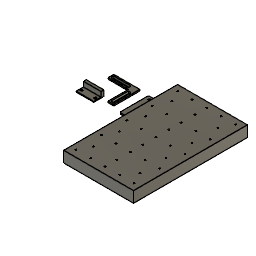
Spoilboard (Autodesk Fusion 360 design; units mm, degrees)
Autodesk Fusion 360 part; units mm, degrees
note: some values were not read from the file. Set by a fixed rule: which sketch regions a step uses.
sketch "Sketch1" plane through (0, 0, 0) normal (0, 1, 0) x (1, 0, 0)
  line L0 (0, 0) -> (60, 0)
  line L1 (60, 0) -> (60, -80)
  line L2 (60, -80) -> (0, -80)
  line L3 (0, -80) -> (0, 0)
  line L4 (40, -80) -> (0, -40)
  line L5 (60, -80) -> (50, -80)
  line L6 (50, -40) -> (60, -40)
  line L7 (60, -40) -> (60, -80)
  circle A0 centre (50, -70) radius 2.5
  circle A1 centre (50, -50) radius 2.5
  line L8 (0, 0) -> (55, 0)
  line L9 (55, 0) -> (55, -10)
  line L10 (55, -10) -> (0, -10)
  line L11 (0, -10) -> (0, 0)
  line L12 (0, 0) -> (55, 0)
  line L13 (55, 0) -> (55, -30)
  line L14 (55, -30) -> (0, -30)
  line L15 (0, -30) -> (0, 0)
  circle A2 centre (20, -30) radius 1.55
  circle A3 centre (40, -30) radius 1.55
  circle A4 centre (20, -10) radius 1.55
  circle A5 centre (40, -10) radius 1.55
  dimension "d1" = 60
  dimension "d2" = 80
  dimension "d3" = 20
  dimension "d4" = 40
  dimension "d5" = 5
  dimension "d6" = 5
  dimension "d7" = 10
  dimension "d8" = 30
  dimension "d9" = 3.1
  dimension "d10" = 3.1
  dimension "d11" = 3.1
  dimension "d12" = 3.1
  dimension "d13" = 20
  dimension "d14" = 20
  dimension "d15" = 20
  dimension "d16" = 20
  constraint horizontal L0
  constraint vertical L1
  constraint horizontal L2
  constraint vertical L3
  constraint coincident L0.start L3.end
  constraint coincident L2 L4.start
  constraint coincident L3 L4.end
  constraint horizontal L5
  constraint horizontal L6
  constraint vertical L7
  constraint horizontal L8
  constraint vertical L9
  constraint horizontal L10
  constraint vertical L11
  constraint horizontal L12
  constraint vertical L13
  constraint horizontal L14
  constraint vertical L15
  constraint coincident L14 A2.centre
  constraint coincident L14 A3.centre
  constraint coincident L10 A4.centre
  constraint coincident L10 A5.centre
  measures "d1" distance of L0.start L0.end
  measures "d2" distance of L0.start L2.end
  measures "d3" distance of L1.end L4.start
  measures "d4" distance of L0 L4.end
  measures "d5" diameter of A0
  measures "d6" diameter of A1
  measures "d7" distance of L0.start L10.end
  measures "d8" distance of L0.start L14.end
  measures "d9" diameter of A2
  measures "d10" diameter of A3
  measures "d11" diameter of A4
  measures "d12" diameter of A5
  measures "d13" distance of L15 A4.centre
  measures "d14" distance of L1 A5.centre
  measures "d15" distance of L1 A3.centre
  measures "d16" distance of L3 A2.centre
extrude "Extrude1" add sketch "Sketch1" against normal blind 10 contours L0 L3 L8 L9 L10 L11 L12 L13 L15 A4 A5 | L0 L1 L2 L3 L4 L5 L7 L9 L13 L14 A2 A3 | L3 L10 L13 L14 L15 A2 A3 A4 A5 makes body 1
sketch "Sketch2" plane through (0, -10, 0) normal (0, -1, 0) x (1, 0, 0)
  circle A0 centre (40, 30) radius 1.55
  circle A1 centre (20, 30) radius 1.55
  circle A2 centre (50, 70) radius 2.5
  circle A3 centre (20, 10) radius 1.55
  circle A4 centre (50, 50) radius 2.5
  circle A5 centre (40, 10) radius 1.55
  line L0 (0, 40) -> (0, 0)
  line L1 (0, 0) -> (60, 0)
  line L2 (60, 0) -> (60, 80)
  line L3 (60, 80) -> (40, 80)
  line L4 (40, 80) -> (0, 40)
  circle A6 centre (20, 30) radius 3
  circle A7 centre (40, 30) radius 3
  circle A8 centre (40, 10) radius 3
  circle A9 centre (20, 10) radius 3
  dimension "d19" = 6
  dimension "d20" = 6
  dimension "d21" = 6
  dimension "d22" = 6
  constraint concentric A1 A6
  constraint concentric A0 A7
  constraint concentric A5 A8
  constraint concentric A3 A9
  measures "d19" diameter of A6
  measures "d20" diameter of A7
  measures "d21" diameter of A8
  measures "d22" diameter of A9
extrude "Extrude2" cut sketch "Sketch2" against normal blind 6.5 contours A6 | A7 | A8 | A9 bodies 1
ref_plane "WorkPlane1" through (-10, -5, 20) normal (-1, 0, 0) x (0, 0, -1)
sketch "Sketch3" plane through (0, 0, 0) normal (0, 0, 1) x (1, 0, 0)
  line L0 (0, 0) -> (241, 0)
  line L1 (241, 0) -> (241, -393)
  line L2 (241, -393) -> (0, -393)
  line L3 (0, -393) -> (0, 0)
  dimension "d30" = 393
  dimension "d31" = 241
  constraint horizontal L0
  constraint vertical L1
  constraint horizontal L2
  constraint vertical L3
  constraint coincident L0.start L3.end
  measures "d30" distance of L0.start L2.end
  measures "d31" distance of L0.start L0.end
extrude "Extrude4" add sketch "Sketch3" along normal blind 38 separate body makes body 2
sketch "Sketch4" plane through (0, 0, 38) normal (0, 0, 1) x (-1, 0, 0)
  line L0 (0, 393) -> (-241, 393)
  line L1 (-241, 393) -> (-241, 0)
  line L2 (-241, 0) -> (0, 0)
  line L3 (0, 0) -> (0, 393)
  point P0 (-220, 20)
  point P1 (-170, 20)
  point P2 (-120, 20)
  point P3 (-70, 20)
  point P4 (-20, 20)
  point P5 (-220, 107.5)
  point P6 (-170, 107.5)
  point P7 (-120, 107.5)
  point P8 (-70, 107.5)
  point P9 (-20, 107.5)
  point P10 (-220, 195)
  point P11 (-170, 195)
  point P12 (-120, 195)
  point P13 (-70, 195)
  point P14 (-20, 195)
  point P15 (-220, 282.5)
  point P16 (-170, 282.5)
  point P17 (-120, 282.5)
  point P18 (-70, 282.5)
  point P19 (-20, 282.5)
  point P20 (-220, 370)
  point P21 (-170, 370)
  point P22 (-120, 370)
  point P23 (-70, 370)
  point P24 (-20, 370)
  point P25 (-200, 60)
  point P26 (-120, 60)
  point P27 (-40, 60)
  point P28 (-200, 150)
  point P29 (-120, 150)
  point P30 (-40, 150)
  point P31 (-200, 240)
  point P32 (-120, 240)
  point P33 (-40, 240)
  point P34 (-200, 330)
  point P35 (-120, 330)
  point P36 (-40, 330)
  dimension "d36" = 200
  dimension "d37" = 350
  dimension "d40" = 160
  dimension "d41" = 270
hole "Hole1" at (70, -370, 38) at (20, -370, 38) at (40, -330, 38) at (120, -370, 38) at (170, -370, 38) at (220, -370, 38) at (200, -330, 38) at (120, -330, 38) at (220, -282.5, 38) at (170, -282.5, 38) at (20, -282.5, 38) at (70, -282.5, 38) at (120, -282.5, 38) at (120, -240, 38) at (200, -240, 38) at (40, -240, 38) at (20, -195, 38) at (70, -195, 38) at (120, -195, 38) at (170, -195, 38) at (220, -195, 38) at (200, -150, 38) at (120, -150, 38) at (40, -150, 38) at (20, -107.5, 38) at (70, -107.5, 38) at (120, -107.5, 38) at (170, -107.5, 38) at (220, -107.5, 38) at (200, -60, 38) at (120, -60, 38) at (40, -60, 38) at (20, -20, 38) at (70, -20, 38) at (120, -20, 38) at (170, -20, 38) at (220, -20, 38) direction (0, 0, -1) diameter 5 depth 38 tip angle 118 bodies 2
sketch "Sketch5" plane through (0, 0, 38) normal (0, 0, 1) x (-1, 0, 0)
  circle A0 centre (-170, 20) radius 2.5
  circle A1 centre (-70, 20) radius 2.5
  circle A2 centre (-40, 60) radius 2.5
  circle A3 centre (-200, 60) radius 2.5
  circle A4 centre (-170, 107.5) radius 2.5
  circle A5 centre (-70, 107.5) radius 2.5
  circle A6 centre (-40, 150) radius 2.5
  circle A7 centre (-200, 150) radius 2.5
  circle A8 centre (-170, 195) radius 2.5
  circle A9 centre (-70, 195) radius 2.5
  circle A10 centre (-40, 240) radius 2.5
  circle A11 centre (-120, 240) radius 2.5
  circle A12 centre (-70, 282.5) radius 2.5
  circle A13 centre (-170, 282.5) radius 2.5
  circle A14 centre (-120, 330) radius 2.5
  circle A15 centre (-220, 370) radius 2.5
  circle A16 centre (-120, 370) radius 2.5
  circle A17 centre (-20, 370) radius 2.5
  circle A18 centre (-70, 370) radius 2.5
  circle A19 centre (-40, 330) radius 2.5
  circle A20 centre (-170, 370) radius 2.5
  circle A21 centre (-200, 330) radius 2.5
  circle A22 centre (-220, 282.5) radius 2.5
  circle A23 centre (-20, 282.5) radius 2.5
  circle A24 centre (-120, 282.5) radius 2.5
  circle A25 centre (-200, 240) radius 2.5
  circle A26 centre (-20, 195) radius 2.5
  circle A27 centre (-120, 195) radius 2.5
  circle A28 centre (-220, 195) radius 2.5
  circle A29 centre (-120, 150) radius 2.5
  circle A30 centre (-20, 107.5) radius 2.5
  circle A31 centre (-120, 107.5) radius 2.5
  circle A32 centre (-220, 107.5) radius 2.5
  circle A33 centre (-120, 60) radius 2.5
  circle A34 centre (-20, 20) radius 2.5
  circle A35 centre (-120, 20) radius 2.5
  circle A36 centre (-220, 20) radius 2.5
  line L0 (0, 393) -> (-241, 393)
  line L1 (-241, 393) -> (-241, 0)
  line L2 (-241, 0) -> (0, 0)
  line L3 (0, 0) -> (0, 393)
  line L4 (80, 100) -> (80, 30)
  line L5 (80, 30) -> (100, 30)
  line L6 (100, 50) -> (100, 120)
  line L7 (100, 120) -> (80, 120)
  line L8 (80, 120) -> (80, 100)
  line L9 (100, 50) -> (170, 50)
  line L10 (100, 30) -> (170, 30)
  line L11 (170, 30) -> (170, 50)
  dimension "d46" = 90
  constraint vertical L4
  constraint perpendicular L4 L5
  constraint perpendicular L5 L6
  constraint perpendicular L6 L7
  constraint perpendicular L7 L8
  constraint perpendicular L6 L9
  constraint perpendicular L6 L10
  constraint perpendicular L10 L11
  measures "d46" distance of L4 L11
sketch "Sketch7" plane through (0, 0, 38) normal (0, 0, 1) x (-1, 0, 0)
  line L0 (85, 115) -> (95, 115)
  line L1 (95, 115) -> (95, 55)
  line L2 (95, 55) -> (85, 55)
  line L3 (85, 55) -> (85, 115)
  line L4 (105, 45) -> (165, 45)
  line L5 (165, 45) -> (165, 35)
  line L6 (165, 35) -> (105, 35)
  line L7 (105, 35) -> (105, 45)
  constraint horizontal L0
  constraint vertical L1
  constraint horizontal L2
  constraint vertical L3
  constraint horizontal L4
  constraint vertical L5
  constraint horizontal L6
  constraint vertical L7
extrude "Extrude9" add sketch "Sketch5" along normal blind 5 separate body contours L4 L5 L6 L7 L8 L9 L10 L11 makes body 3
extrude "Extrude10" cut sketch "Sketch7" along normal blind 20 bodies 3
draft "Draft1" angle 30 neutral plane through (0, 0, 43) pull (0, 0, 1) 8 faces at (-85, -75, 39.6667) (-105, -38.3333, 39.6667) (-95, -95, 39.6667) (-165, -41.6667, 39.6667) (-88.3333, -115, 39.6667) (-125, -45, 39.6667) (-145, -35, 39.6667) (-91.6667, -55, 39.6667) on bodies 3
move_body "Move7" bodies 3 to x (1, 0, 0) y (0, 1, 0) z (0, 0, 1) at (0, -20, -34.641)
sketch "Sketch8" plane through (0, 0, 0) normal (0, 0, 1) x (1, 0, 0)
  line L0 (-45, -50) -> (-25, -50)
  line L1 (-20, -55) -> (-20, -61.8388)
  line L2 (-37.6229, -150) -> (-45, -150)
  line L3 (-50, -145) -> (-50, -55)
  spline S0 degree 5 poles (-22.4081, -66.1145) (-22.6473, -66.2595) (-23.5601, -66.8506) (-25.0379, -68.0682) (-26.8635, -70.273) (-28.7085, -74.0094) (-30.1195, -79.4806) (-30.8706, -86.0261) (-31.077, -93.4328) (-30.8971, -101.4083) (-30.5136, -109.6167) (-30.1163, -117.7095) (-29.8841, -125.3579) (-29.9696, -132.2821) (-30.4781, -138.2915) (-31.2767, -142.3725) (-32.1097, -144.9675) (-32.7761, -146.499) (-33.1491, -147.2333) (-33.1747, -147.2833) knots 0.043571 0.043571 0.043571 0.043571 0.043571 0.043571 0.066667 0.133333 0.2 0.266667 0.333333 0.4 0.466667 0.533333 0.6 0.666667 0.733333 0.8 0.866667 0.933333 0.938232 0.938232 0.938232 0.938232 0.938232 0.938232
  arc A0 (-50, -145) -> (-45, -150) centre (-45, -145) ccw
  arc A1 (-37.6229, -150) -> (-33.1747, -147.2833) centre (-37.6229, -145) ccw
  arc A2 (-22.4081, -66.1145) -> (-20, -61.8388) centre (-25, -61.8388) ccw
  arc A3 (-20, -55) -> (-25, -50) centre (-25, -55) ccw
  arc A4 (-45, -50) -> (-50, -55) centre (-45, -55) ccw
  circle A5 centre (-36.5, -62) radius 2.5
  point P0 (-30, -80)
  point P1 (-30, -130)
  dimension "d61" = 5
  dimension "d62" = 5
  constraint horizontal L0
  constraint vertical L1
  constraint horizontal L2
  constraint vertical L3
  constraint tangent L2 A0
  constraint tangent L3 A0
  constraint tangent S0 A1
  constraint tangent L2 A1
  constraint equal A0 A1
  constraint tangent S0 A2
  constraint tangent L1 A2
  constraint equal A0 A2
  constraint tangent L0 A3
  constraint tangent L1 A3
  constraint equal A0 A3
  constraint tangent L0 A4
  constraint tangent L3 A4
  constraint equal A0 A4
  measures "d61" radius of A0
  measures "d62" diameter of A5
extrude "Extrude11" add sketch "Sketch8" along normal blind 5 separate body makes body 4
sketch "Sketch9" plane through (0, 0, 5) normal (0, 0, 1) x (-1, 0, 0)
  circle A0 centre (36.5, 62) radius 2.5
  arc A1 (20, 55) -> (25, 50) centre (25, 55) ccw
  line L0 (25, 50) -> (45, 50)
  arc A2 (45, 50) -> (50, 55) centre (45, 55) ccw
  line L1 (50, 55) -> (50, 145)
  arc A3 (50, 145) -> (45, 150) centre (45, 145) ccw
  line L2 (45, 150) -> (37.6229, 150)
  arc A4 (37.6229, 150) -> (33.1747, 147.2833) centre (37.6229, 145) ccw
  spline S0 degree 5 poles (33.1747, 147.2833) (33.1491, 147.2333) (32.7761, 146.499) (32.1097, 144.9675) (31.2767, 142.3725) (30.4781, 138.2915) (29.9696, 132.2821) (29.8841, 125.3579) (30.1163, 117.7095) (30.5136, 109.6167) (30.8971, 101.4083) (31.077, 93.4328) (30.8706, 86.0261) (30.1195, 79.4806) (28.7085, 74.0094) (26.8635, 70.273) (25.0379, 68.0682) (23.5601, 66.8506) (22.6473, 66.2595) (22.4081, 66.1145) knots -0.938232 -0.938232 -0.938232 -0.938232 -0.938232 -0.938232 -0.933333 -0.866667 -0.8 -0.733333 -0.666667 -0.6 -0.533333 -0.466667 -0.4 -0.333333 -0.266667 -0.2 -0.133333 -0.066667 -0.043571 -0.043571 -0.043571 -0.043571 -0.043571 -0.043571
  arc A5 (22.4081, 66.1145) -> (20, 61.8388) centre (25, 61.8388) ccw
  line L3 (20, 61.8388) -> (20, 55)
  circle A6 centre (36.5, 62.0016) radius 3.5
  dimension "d65" = 7
  measures "d65" diameter of A6
extrude "Extrude12" cut sketch "Sketch9" against normal blind 2.5 contours A6 bodies 4
sketch "Sketch10" plane through (0, 0, 0) normal (0, 0, 1) x (1, 0, 0)
  line L0 (-135, -160) -> (-190, -160)
  line L1 (-190, -160) -> (-190, -125)
  line L2 (-190, -125) -> (-135, -125)
  line L3 (-135, -125) -> (-135, -160)
  line L4 (-135, -135) -> (-190, -135)
  line L5 (-190, -135) -> (-190, -160)
  line L6 (-190, -160) -> (-135, -160)
  line L7 (-135, -160) -> (-135, -135)
  constraint horizontal L0
  constraint vertical L1
  constraint horizontal L2
  constraint vertical L3
  constraint horizontal L4
  constraint vertical L5
  constraint horizontal L6
  constraint vertical L7
  constraint coincident L3 L4.start
extrude "Extrude13" add sketch "Sketch10" along normal blind 3 separate body contours L0 L1 L3 L4 L5 L6 L7 makes body 5
extrude "Extrude14" add sketch "Sketch10" along normal blind 15 contours L1 L2 L3 L4 bodies 5
sketch "Sketch11" plane through (0, 0, 3) normal (0, 0, 1) x (-1, 0, 0)
  line L0 (135, 160) -> (135, 135)
  line L1 (135, 135) -> (190, 135)
  line L2 (190, 135) -> (190, 160)
  line L3 (190, 160) -> (135, 160)
  circle A0 centre (184, 147) radius 3.5
  circle A1 centre (184, 147) radius 2.5
  circle A2 centre (136.5001, 146.9246) radius 3.5
  circle A3 centre (136.5001, 146.9246) radius 2.5
  dimension "d73" = 7
  dimension "d74" = 5
  dimension "d75" = 7
  dimension "d76" = 5
  dimension "d78" = 47.5
  constraint concentric A2 A3
  constraint concentric A0 A1
  measures "d73" diameter of A0
  measures "d74" diameter of A1
  measures "d75" diameter of A2
  measures "d76" diameter of A3
  measures "d78" distance of A0.centre A2.centre
extrude "Extrude15" add 1 faces at (-135, -128.3333, 6) along direction (1, 0, 0) blind 6 on bodies 5 bodies 5
extrude "Extrude16" cut sketch "Sketch11" against normal blind 1 contours L0 A2 A3 | L0 A2 A3 | A0 bodies 5
extrude "Extrude17" cut 2 faces at (-135.7493, -146.563, 3) (-183.2947, -146.7544, 3) along direction (0, 0, -1) blind 5 on bodies 5 bodies 5
extrude "Extrude18" add 1 faces at (-149.3333, -131.6667, 15) along direction (0, 0, 1) blind 5 on bodies 5 bodies 5
sketch "Sketch6" plane through (0, 0, 38) normal (0, 0, 1) x (-1, 0, 0)
  line L0 (85, 115) -> (90, 115)
  line L1 (90, 115) -> (90, 55)
  line L2 (90, 55) -> (85, 55)
  line L3 (85, 55) -> (85, 115)
  line L4 (100, 40) -> (165, 40)
  line L5 (165, 40) -> (165, 35)
  line L6 (165, 35) -> (100, 35)
  line L7 (100, 35) -> (100, 40)
  constraint horizontal L0
  constraint vertical L1
  constraint horizontal L2
  constraint vertical L3
  constraint horizontal L4
  constraint vertical L5
  constraint horizontal L6
  constraint vertical L7
extrude "Extrude7" [suppressed]
extrude "Extrude8" [suppressed]
extrude "Extrude6" [suppressed]
extrude "Extrude5" [suppressed]
hidden bodies 1
equation "d23 = -10.00 mm + 3.5 mm"
